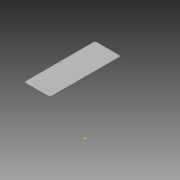
# Autodesk Inventor part: Base
Saved by Autodesk Inventor 2015 (Build 190159000, 159)
## iProperties
Created: 2014-07-24
Part Number: Base
Material: Generic
Document SubType Name: Modeling
Designer: Michael
Density: 1 g/cm^3
Appearance: Default
Author: Michael
Autodesk Inventor part; units mm, degrees
(part 1 of 2)
ref_plane "YZ Plane" through (0, 0, 0) normal (1, 0, 0) x (0, 1, 0)
ref_plane "XZ Plane" through (0, 0, 0) normal (0, 1, 0) x (-1, 0, 0)
ref_plane "XY Plane" through (0, 0, 0) normal (0, 0, 1) x (1, 0, 0)
sketch "Sketch1" plane through (0, 0, 0) normal (0, 1, 0) x (-1, 0, 0)
  circle A0 centre (194.2191, -316.0168) radius 1.4732
  circle A1 centre (279.9441, -316.0168) radius 1.4732
  circle A2 centre (279.9441, -192.1918) radius 1.4732
  circle A3 centre (194.2191, -192.1918) radius 1.4732
  circle A4 centre (194.2191, -68.3668) radius 1.4732
  circle A5 centre (279.9441, -68.3668) radius 1.4732
  arc A6 (191.0441, -316.0168) -> (194.2191, -319.1918) centre (194.2191, -316.0168) ccw
  arc A7 (279.9441, -319.1918) -> (283.1191, -316.0168) centre (279.9441, -316.0168) ccw
  arc A8 (194.2191, -65.1918) -> (191.0441, -68.3668) centre (194.2191, -68.3668) ccw
  arc A9 (283.1191, -68.3668) -> (279.9441, -65.1918) centre (279.9441, -68.3668) ccw
  line L0 (194.2191, -65.1918) -> (279.9441, -65.1918)
  line L1 (191.0441, -316.0168) -> (191.0441, -68.3668)
  line L2 (279.9441, -319.1918) -> (194.2191, -319.1918)
  line L3 (283.1191, -68.3668) -> (283.1191, -316.0168)
  circle A10 centre (95.0063, -316.0168) radius 1.4732
  circle A11 centre (180.7313, -316.0168) radius 1.4732
  circle A12 centre (180.7313, -192.1918) radius 1.4732
  circle A13 centre (95.0063, -192.1918) radius 1.4732
  circle A14 centre (95.0063, -68.3668) radius 1.4732
  circle A15 centre (180.7313, -68.3668) radius 1.4732
  arc A16 (91.8313, -316.0168) -> (95.0063, -319.1918) centre (95.0063, -316.0168) ccw
  arc A17 (180.7313, -319.1918) -> (183.9063, -316.0168) centre (180.7313, -316.0168) ccw
  line L4 (183.9063, -312.8418) -> (183.9063, -316.0168)
  line L5 (180.7313, -319.1918) -> (177.5563, -319.1918)
  arc A18 (95.0063, -65.1918) -> (91.8313, -68.3668) centre (95.0063, -68.3668) ccw
  line L6 (91.8313, -71.5418) -> (91.8313, -68.3668)
  line L7 (95.0063, -65.1918) -> (98.1813, -65.1918)
  arc A19 (183.9063, -68.3668) -> (180.7313, -65.1918) centre (180.7313, -68.3668) ccw
  line L8 (98.1813, -319.1918) -> (95.0063, -319.1918)
  line L9 (91.8313, -316.0168) -> (91.8313, -312.8418)
  line L10 (95.0063, -65.1918) -> (180.7313, -65.1918)
  line L11 (91.8313, -316.0168) -> (91.8313, -68.3668)
  line L12 (180.7313, -319.1918) -> (95.0063, -319.1918)
  line L13 (183.9063, -68.3668) -> (183.9063, -316.0168)
  line L14 (115.5168, -195.2716) -> (114.9834, -195.2716)
  line L15 (114.9834, -195.2716) -> (114.9834, -193.5952)
  line L16 (114.9834, -193.5952) -> (111.5798, -193.5952)
  line L17 (111.5798, -193.5952) -> (111.5798, -192.7062)
  line L18 (111.5798, -192.7062) -> (108.7858, -192.7062)
  line L19 (108.7858, -192.7062) -> (108.7858, -193.5952)
  line L20 (108.7858, -193.5952) -> (102.6898, -193.5952)
  line L21 (102.6898, -193.5952) -> (102.6898, -195.2716)
  line L22 (102.6898, -195.2716) -> (101.5468, -195.2716)
  line L23 (101.5468, -195.2716) -> (101.5468, -198.5736)
  line L24 (101.5468, -198.5736) -> (102.6898, -198.5736)
  line L25 (102.6898, -198.5736) -> (102.6898, -200.25)
  line L26 (102.6898, -200.25) -> (108.7858, -200.25)
  line L27 (108.7858, -200.25) -> (108.7858, -201.8756)
  line L28 (108.7858, -201.8756) -> (106.7894, -201.8756)
  line L29 (106.7894, -201.8756) -> (106.7894, -201.0628)
  line L30 (106.7894, -201.0628) -> (103.4772, -201.0628)
  line L31 (103.4772, -201.0628) -> (103.4772, -201.8756)
  line L32 (102.3088, -201.8756) -> (103.4772, -201.8756)
  line L33 (102.3088, -201.8756) -> (102.3088, -215.8456)
  line L34 (102.3088, -215.8456) -> (103.4772, -215.8456)
  line L35 (103.4772, -215.8456) -> (103.4772, -216.6584)
  line L36 (103.4772, -216.6584) -> (106.7894, -216.6584)
  line L37 (106.7894, -216.6584) -> (106.7894, -215.8456)
  line L38 (106.7894, -215.8456) -> (108.7858, -215.8456)
  line L39 (108.7858, -215.8456) -> (108.7858, -217.4712)
  line L40 (108.7858, -217.4712) -> (102.6898, -217.4712)
  line L41 (102.6898, -217.4712) -> (102.6898, -219.1476)
  line L42 (102.6898, -219.1476) -> (101.5468, -219.1476)
  line L43 (101.5468, -219.1476) -> (101.5468, -222.4496)
  line L44 (101.5468, -222.4496) -> (102.6898, -222.4496)
  line L45 (102.6898, -222.4496) -> (102.6898, -224.126)
  line L46 (102.6898, -224.126) -> (108.7858, -224.126)
  line L47 (108.7858, -224.126) -> (108.7858, -225.015)
  line L48 (108.7858, -225.015) -> (111.5798, -225.015)
  line L49 (111.5798, -225.015) -> (111.5798, -224.126)
  line L50 (111.5798, -224.126) -> (114.9834, -224.126)
  line L51 (114.9834, -224.126) -> (114.9834, -222.4496)
  line L52 (114.9834, -222.4496) -> (115.5168, -222.4496)
  line L53 (115.5168, -222.4496) -> (115.5168, -219.1476)
  line L54 (115.5168, -219.1476) -> (114.9834, -219.1476)
  line L55 (114.9834, -219.1476) -> (114.9834, -217.4712)
  line L56 (114.9834, -217.4712) -> (111.5798, -217.4712)
  line L57 (111.5798, -217.4712) -> (111.5798, -216.6584)
  line L58 (111.5798, -216.6584) -> (115.2984, -216.6584)
  line L59 (115.2984, -216.6584) -> (115.2984, -215.8456)
  line L60 (115.2984, -215.8456) -> (116.2788, -215.8456)
  line L61 (116.2788, -215.8456) -> (116.2788, -201.8756)
  line L62 (116.2788, -201.8756) -> (115.2984, -201.8756)
  line L63 (115.2984, -201.8756) -> (115.2984, -201.0628)
  line L64 (115.2984, -201.0628) -> (111.5798, -201.0628)
  line L65 (111.5798, -201.0628) -> (111.5798, -200.25)
  line L66 (111.5798, -200.25) -> (114.9834, -200.25)
  line L67 (114.9834, -200.25) -> (114.9834, -198.5736)
  line L68 (114.9834, -198.5736) -> (115.5168, -198.5736)
  line L69 (115.5168, -198.5736) -> (115.5168, -195.2716)
  line L70 (115.5168, -152.4091) -> (114.9834, -152.4091)
  line L71 (114.9834, -152.4091) -> (114.9834, -150.7327)
  line L72 (114.9834, -150.7327) -> (111.5798, -150.7327)
  line L73 (111.5798, -150.7327) -> (111.5798, -149.8437)
  line L74 (111.5798, -149.8437) -> (108.7858, -149.8437)
  line L75 (108.7858, -149.8437) -> (108.7858, -150.7327)
  line L76 (108.7858, -150.7327) -> (102.6898, -150.7327)
  line L77 (102.6898, -150.7327) -> (102.6898, -152.4091)
  line L78 (102.6898, -152.4091) -> (101.5468, -152.4091)
  line L79 (101.5468, -152.4091) -> (101.5468, -155.7111)
  line L80 (101.5468, -155.7111) -> (102.6898, -155.7111)
  line L81 (102.6898, -155.7111) -> (102.6898, -157.3875)
  line L82 (102.6898, -157.3875) -> (108.7858, -157.3875)
  line L83 (108.7858, -157.3875) -> (108.7858, -159.0131)
  line L84 (108.7858, -159.0131) -> (106.7894, -159.0131)
  line L85 (106.7894, -159.0131) -> (106.7894, -158.2003)
  line L86 (106.7894, -158.2003) -> (103.4772, -158.2003)
  line L87 (103.4772, -158.2003) -> (103.4772, -159.0131)
  line L88 (102.3088, -159.0131) -> (103.4772, -159.0131)
  line L89 (102.3088, -159.0131) -> (102.3088, -172.9831)
  line L90 (102.3088, -172.9831) -> (103.4772, -172.9831)
  line L91 (103.4772, -172.9831) -> (103.4772, -173.7959)
  line L92 (103.4772, -173.7959) -> (106.7894, -173.7959)
  line L93 (106.7894, -173.7959) -> (106.7894, -172.9831)
  line L94 (106.7894, -172.9831) -> (108.7858, -172.9831)
  line L95 (108.7858, -172.9831) -> (108.7858, -174.6087)
  line L96 (108.7858, -174.6087) -> (102.6898, -174.6087)
  line L97 (102.6898, -174.6087) -> (102.6898, -176.2851)
  line L98 (102.6898, -176.2851) -> (101.5468, -176.2851)
  line L99 (101.5468, -176.2851) -> (101.5468, -179.5871)
  line L100 (101.5468, -179.5871) -> (102.6898, -179.5871)
  line L101 (102.6898, -179.5871) -> (102.6898, -181.2635)
  line L102 (102.6898, -181.2635) -> (108.7858, -181.2635)
  line L103 (108.7858, -181.2635) -> (108.7858, -182.1525)
  line L104 (108.7858, -182.1525) -> (111.5798, -182.1525)
  line L105 (111.5798, -182.1525) -> (111.5798, -181.2635)
  line L106 (111.5798, -181.2635) -> (114.9834, -181.2635)
  line L107 (114.9834, -181.2635) -> (114.9834, -179.5871)
  line L108 (114.9834, -179.5871) -> (115.5168, -179.5871)
  line L109 (115.5168, -179.5871) -> (115.5168, -176.2851)
  line L110 (115.5168, -176.2851) -> (114.9834, -176.2851)
  line L111 (114.9834, -176.2851) -> (114.9834, -174.6087)
  line L112 (114.9834, -174.6087) -> (111.5798, -174.6087)
  line L113 (111.5798, -174.6087) -> (111.5798, -173.7959)
  line L114 (111.5798, -173.7959) -> (115.2984, -173.7959)
  line L115 (115.2984, -173.7959) -> (115.2984, -172.9831)
  line L116 (115.2984, -172.9831) -> (116.2788, -172.9831)
  line L117 (116.2788, -172.9831) -> (116.2788, -159.0131)
  line L118 (116.2788, -159.0131) -> (115.2984, -159.0131)
  line L119 (115.2984, -159.0131) -> (115.2984, -158.2003)
  line L120 (115.2984, -158.2003) -> (111.5798, -158.2003)
  line L121 (111.5798, -158.2003) -> (111.5798, -157.3875)
  line L122 (111.5798, -157.3875) -> (114.9834, -157.3875)
  line L123 (114.9834, -157.3875) -> (114.9834, -155.7111)
  line L124 (114.9834, -155.7111) -> (115.5168, -155.7111)
  line L125 (115.5168, -155.7111) -> (115.5168, -152.4091)
  line L126 (111.7982, -274.8815) -> (115.2983, -274.8815)
  line L127 (115.2983, -290.4771) -> (111.7982, -290.4771)
  line L128 (106.7893, -290.4771) -> (103.2892, -290.4771)
  line L129 (103.2892, -274.8815) -> (106.7893, -274.8815)
  line L130 (111.7982, -274.8815) -> (111.7982, -275.6943)
  line L131 (111.7982, -289.6643) -> (111.7982, -290.4771)
  line L132 (106.7893, -290.4771) -> (106.7893, -289.6643)
  line L133 (106.7893, -275.6943) -> (106.7893, -274.8815)
  line L134 (106.7893, -289.6643) -> (106.7893, -290.4771)
  line L135 (106.7893, -290.4771) -> (103.2892, -290.4771)
  line L136 (103.2892, -290.4771) -> (103.2892, -289.6643)
  line L137 (103.2892, -275.6943) -> (103.2892, -274.8815)
  line L138 (103.2892, -274.8815) -> (106.7893, -274.8815)
  line L139 (106.7893, -274.8815) -> (106.7893, -275.6943)
  line L140 (111.7982, -275.6943) -> (111.7982, -274.8815)
  line L141 (111.7982, -274.8815) -> (115.2983, -274.8815)
  line L142 (115.2983, -274.8815) -> (115.2983, -275.6943)
  line L143 (115.2983, -289.6643) -> (115.2983, -290.4771)
  line L144 (115.2983, -290.4771) -> (111.7982, -290.4771)
  line L145 (111.7982, -290.4771) -> (111.7982, -289.6643)
  line L146 (115.2983, -275.6943) -> (116.2788, -275.6943)
  line L147 (116.2788, -275.6943) -> (116.2788, -289.6643)
  line L148 (116.2788, -289.6643) -> (115.2983, -289.6643)
  line L149 (111.7982, -289.6643) -> (106.7893, -289.6643)
  line L150 (103.2892, -289.6643) -> (102.3088, -289.6643)
  line L151 (102.3088, -289.6643) -> (102.3088, -275.6943)
  line L152 (102.3088, -275.6943) -> (103.2892, -275.6943)
  line L153 (106.7893, -275.6943) -> (111.7982, -275.6943)
  line L154 (111.7982, -293.9315) -> (115.2983, -293.9315)
  line L155 (115.2983, -309.5271) -> (111.7982, -309.5271)
  line L156 (106.7893, -309.5271) -> (103.2892, -309.5271)
  line L157 (103.2892, -293.9315) -> (106.7893, -293.9315)
  line L158 (111.7982, -293.9315) -> (111.7982, -294.7443)
  line L159 (111.7982, -308.7143) -> (111.7982, -309.5271)
  line L160 (106.7893, -309.5271) -> (106.7893, -308.7143)
  line L161 (106.7893, -294.7443) -> (106.7893, -293.9315)
  line L162 (106.7893, -308.7143) -> (106.7893, -309.5271)
  line L163 (106.7893, -309.5271) -> (103.2892, -309.5271)
  line L164 (103.2892, -309.5271) -> (103.2892, -308.7143)
  line L165 (103.2892, -294.7443) -> (103.2892, -293.9315)
  line L166 (103.2892, -293.9315) -> (106.7893, -293.9315)
  line L167 (106.7893, -293.9315) -> (106.7893, -294.7443)
  line L168 (111.7982, -294.7443) -> (111.7982, -293.9315)
  line L169 (111.7982, -293.9315) -> (115.2983, -293.9315)
  line L170 (115.2983, -293.9315) -> (115.2983, -294.7443)
  line L171 (115.2983, -308.7143) -> (115.2983, -309.5271)
  line L172 (115.2983, -309.5271) -> (111.7982, -309.5271)
  line L173 (111.7982, -309.5271) -> (111.7982, -308.7143)
  line L174 (115.2983, -294.7443) -> (116.2788, -294.7443)
  line L175 (116.2788, -294.7443) -> (116.2788, -308.7143)
  line L176 (116.2788, -308.7143) -> (115.2983, -308.7143)
  line L177 (111.7982, -308.7143) -> (106.7893, -308.7143)
  line L178 (103.2892, -308.7143) -> (102.3088, -308.7143)
  line L179 (102.3088, -308.7143) -> (102.3088, -294.7443)
  line L180 (102.3088, -294.7443) -> (103.2892, -294.7443)
  line L181 (106.7893, -294.7443) -> (111.7982, -294.7443)
  line L182 (111.7982, -255.8315) -> (115.2983, -255.8315)
  line L183 (115.2983, -271.4271) -> (111.7982, -271.4271)
  line L184 (106.7893, -271.4271) -> (103.2892, -271.4271)
  line L185 (103.2892, -255.8315) -> (106.7893, -255.8315)
  line L186 (111.7982, -255.8315) -> (111.7982, -256.6443)
  line L187 (111.7982, -270.6143) -> (111.7982, -271.4271)
  line L188 (106.7893, -271.4271) -> (106.7893, -270.6143)
  line L189 (106.7893, -256.6443) -> (106.7893, -255.8315)
  line L190 (106.7893, -270.6143) -> (106.7893, -271.4271)
  line L191 (106.7893, -271.4271) -> (103.2892, -271.4271)
  line L192 (103.2892, -271.4271) -> (103.2892, -270.6143)
  line L193 (103.2892, -256.6443) -> (103.2892, -255.8315)
  line L194 (103.2892, -255.8315) -> (106.7893, -255.8315)
  line L195 (106.7893, -255.8315) -> (106.7893, -256.6443)
  line L196 (111.7982, -256.6443) -> (111.7982, -255.8315)
  line L197 (111.7982, -255.8315) -> (115.2983, -255.8315)
  line L198 (115.2983, -255.8315) -> (115.2983, -256.6443)
  line L199 (115.2983, -270.6143) -> (115.2983, -271.4271)
  line L200 (115.2983, -271.4271) -> (111.7982, -271.4271)
  line L201 (111.7982, -271.4271) -> (111.7982, -270.6143)
  line L202 (115.2983, -256.6443) -> (116.2788, -256.6443)
  line L203 (116.2788, -256.6443) -> (116.2788, -270.6143)
  line L204 (116.2788, -270.6143) -> (115.2983, -270.6143)
  line L205 (111.7982, -270.6143) -> (106.7893, -270.6143)
  line L206 (103.2892, -270.6143) -> (102.3088, -270.6143)
  line L207 (102.3088, -270.6143) -> (102.3088, -256.6443)
  line L208 (102.3088, -256.6443) -> (103.2892, -256.6443)
  line L209 (106.7893, -256.6443) -> (111.7982, -256.6443)
  line L210 (111.7982, -234.4003) -> (115.2983, -234.4003)
  line L211 (115.2983, -249.9959) -> (111.7982, -249.9959)
  line L212 (106.7893, -249.9959) -> (103.2892, -249.9959)
  line L213 (103.2892, -234.4003) -> (106.7893, -234.4003)
  line L214 (111.7982, -234.4003) -> (111.7982, -235.2131)
  line L215 (111.7982, -249.1831) -> (111.7982, -249.9959)
  line L216 (106.7893, -249.9959) -> (106.7893, -249.1831)
  line L217 (106.7893, -235.2131) -> (106.7893, -234.4003)
  line L218 (106.7893, -249.1831) -> (106.7893, -249.9959)
  line L219 (106.7893, -249.9959) -> (103.2892, -249.9959)
  line L220 (103.2892, -249.9959) -> (103.2892, -249.1831)
  line L221 (103.2892, -235.2131) -> (103.2892, -234.4003)
  line L222 (103.2892, -234.4003) -> (106.7893, -234.4003)
  line L223 (106.7893, -234.4003) -> (106.7893, -235.2131)
  line L224 (111.7982, -235.2131) -> (111.7982, -234.4003)
  line L225 (111.7982, -234.4003) -> (115.2983, -234.4003)
  line L226 (115.2983, -234.4003) -> (115.2983, -235.2131)
  line L227 (115.2983, -249.1831) -> (115.2983, -249.9959)
  line L228 (115.2983, -249.9959) -> (111.7982, -249.9959)
  line L229 (111.7982, -249.9959) -> (111.7982, -249.1831)
  line L230 (115.2983, -235.2131) -> (116.2788, -235.2131)
  line L231 (116.2788, -235.2131) -> (116.2788, -249.1831)
  line L232 (116.2788, -249.1831) -> (115.2983, -249.1831)
  line L233 (111.7982, -249.1831) -> (106.7893, -249.1831)
  line L234 (103.2892, -249.1831) -> (102.3088, -249.1831)
  line L235 (102.3088, -249.1831) -> (102.3088, -235.2131)
  line L236 (102.3088, -235.2131) -> (103.2892, -235.2131)
  line L237 (106.7893, -235.2131) -> (111.7982, -235.2131)
  line L238 (111.7982, -101.0503) -> (115.2983, -101.0503)
  line L239 (115.2983, -116.6459) -> (111.7982, -116.6459)
  line L240 (106.7893, -116.6459) -> (103.2892, -116.6459)
  line L241 (103.2892, -101.0503) -> (106.7893, -101.0503)
  line L242 (111.7982, -101.0503) -> (111.7982, -101.8631)
  line L243 (111.7982, -115.8331) -> (111.7982, -116.6459)
  line L244 (106.7893, -116.6459) -> (106.7893, -115.8331)
  line L245 (106.7893, -101.8631) -> (106.7893, -101.0503)
  line L246 (106.7893, -115.8331) -> (106.7893, -116.6459)
  line L247 (106.7893, -116.6459) -> (103.2892, -116.6459)
  line L248 (103.2892, -116.6459) -> (103.2892, -115.8331)
  line L249 (103.2892, -101.8631) -> (103.2892, -101.0503)
  line L250 (103.2892, -101.0503) -> (106.7893, -101.0503)
  line L251 (106.7893, -101.0503) -> (106.7893, -101.8631)
  line L252 (111.7982, -101.8631) -> (111.7982, -101.0503)
  line L253 (111.7982, -101.0503) -> (115.2983, -101.0503)
  line L254 (115.2983, -101.0503) -> (115.2983, -101.8631)
  line L255 (115.2983, -115.8331) -> (115.2983, -116.6459)
  line L256 (115.2983, -116.6459) -> (111.7982, -116.6459)
  line L257 (111.7982, -116.6459) -> (111.7982, -115.8331)
  line L258 (115.2983, -101.8631) -> (116.2788, -101.8631)
  line L259 (116.2788, -101.8631) -> (116.2788, -115.8331)
  line L260 (116.2788, -115.8331) -> (115.2983, -115.8331)
  line L261 (111.7982, -115.8331) -> (106.7893, -115.8331)
  line L262 (103.2892, -115.8331) -> (102.3088, -115.8331)
  line L263 (102.3088, -115.8331) -> (102.3088, -101.8631)
  line L264 (102.3088, -101.8631) -> (103.2892, -101.8631)
  line L265 (106.7893, -101.8631) -> (111.7982, -101.8631)
  line L266 (111.7982, -124.8628) -> (115.2983, -124.8628)
  line L267 (115.2983, -140.4584) -> (111.7982, -140.4584)
  line L268 (106.7893, -140.4584) -> (103.2892, -140.4584)
  line L269 (103.2892, -124.8628) -> (106.7893, -124.8628)
  line L270 (111.7982, -124.8628) -> (111.7982, -125.6756)
  line L271 (111.7982, -139.6456) -> (111.7982, -140.4584)
  line L272 (106.7893, -140.4584) -> (106.7893, -139.6456)
  line L273 (106.7893, -125.6756) -> (106.7893, -124.8628)
  line L274 (106.7893, -139.6456) -> (106.7893, -140.4584)
  line L275 (106.7893, -140.4584) -> (103.2892, -140.4584)
  line L276 (103.2892, -140.4584) -> (103.2892, -139.6456)
  line L277 (103.2892, -125.6756) -> (103.2892, -124.8628)
  line L278 (103.2892, -124.8628) -> (106.7893, -124.8628)
  line L279 (106.7893, -124.8628) -> (106.7893, -125.6756)
  line L280 (111.7982, -125.6756) -> (111.7982, -124.8628)
  line L281 (111.7982, -124.8628) -> (115.2983, -124.8628)
  line L282 (115.2983, -124.8628) -> (115.2983, -125.6756)
  line L283 (115.2983, -139.6456) -> (115.2983, -140.4584)
  line L284 (115.2983, -140.4584) -> (111.7982, -140.4584)
  line L285 (111.7982, -140.4584) -> (111.7982, -139.6456)
  line L286 (115.2983, -125.6756) -> (116.2788, -125.6756)
  line L287 (116.2788, -125.6756) -> (116.2788, -139.6456)
  line L288 (116.2788, -139.6456) -> (115.2983, -139.6456)
  line L289 (111.7982, -139.6456) -> (106.7893, -139.6456)
  line L290 (103.2892, -139.6456) -> (102.3088, -139.6456)
  line L291 (102.3088, -139.6456) -> (102.3088, -125.6756)
  line L292 (102.3088, -125.6756) -> (103.2892, -125.6756)
  line L293 (106.7893, -125.6756) -> (111.7982, -125.6756)
  line L294 (111.7982, -77.2378) -> (115.2983, -77.2378)
  line L295 (115.2983, -92.8334) -> (111.7982, -92.8334)
  line L296 (106.7893, -92.8334) -> (103.2892, -92.8334)
  line L297 (103.2892, -77.2378) -> (106.7893, -77.2378)
  line L298 (111.7982, -77.2378) -> (111.7982, -78.0506)
  line L299 (111.7982, -92.0206) -> (111.7982, -92.8334)
  line L300 (106.7893, -92.8334) -> (106.7893, -92.0206)
  line L301 (106.7893, -78.0506) -> (106.7893, -77.2378)
  line L302 (106.7893, -92.0206) -> (106.7893, -92.8334)
  line L303 (106.7893, -92.8334) -> (103.2892, -92.8334)
  line L304 (103.2892, -92.8334) -> (103.2892, -92.0206)
  line L305 (103.2892, -78.0506) -> (103.2892, -77.2378)
  line L306 (103.2892, -77.2378) -> (106.7893, -77.2378)
  line L307 (106.7893, -77.2378) -> (106.7893, -78.0506)
  line L308 (111.7982, -78.0506) -> (111.7982, -77.2378)
  line L309 (111.7982, -77.2378) -> (115.2983, -77.2378)
  line L310 (115.2983, -77.2378) -> (115.2983, -78.0506)
  line L311 (115.2983, -92.0206) -> (115.2983, -92.8334)
  line L312 (115.2983, -92.8334) -> (111.7982, -92.8334)
  line L313 (111.7982, -92.8334) -> (111.7982, -92.0206)
  line L314 (115.2983, -78.0506) -> (116.2788, -78.0506)
  line L315 (116.2788, -78.0506) -> (116.2788, -92.0206)
  line L316 (116.2788, -92.0206) -> (115.2983, -92.0206)
  line L317 (111.7982, -92.0206) -> (106.7893, -92.0206)
  line L318 (103.2892, -92.0206) -> (102.3088, -92.0206)
  line L319 (102.3088, -92.0206) -> (102.3088, -78.0506)
  line L320 (102.3088, -78.0506) -> (103.2892, -78.0506)
  line L321 (106.7893, -78.0506) -> (111.7982, -78.0506)
  line L322 (130.8482, -122.4815) -> (134.3483, -122.4815)
  line L323 (134.3483, -138.0771) -> (130.8482, -138.0771)
  line L324 (125.8393, -138.0771) -> (122.3392, -138.0771)
  line L325 (122.3392, -122.4815) -> (125.8393, -122.4815)
  line L326 (130.8482, -122.4815) -> (130.8482, -123.2943)
  line L327 (130.8482, -137.2643) -> (130.8482, -138.0771)
  line L328 (125.8393, -138.0771) -> (125.8393, -137.2643)
  line L329 (125.8393, -123.2943) -> (125.8393, -122.4815)
  line L330 (125.8393, -137.2643) -> (125.8393, -138.0771)
  line L331 (125.8393, -138.0771) -> (122.3392, -138.0771)
  line L332 (122.3392, -138.0771) -> (122.3392, -137.2643)
  line L333 (122.3392, -123.2943) -> (122.3392, -122.4815)
  line L334 (122.3392, -122.4815) -> (125.8393, -122.4815)
  line L335 (125.8393, -122.4815) -> (125.8393, -123.2943)
  line L336 (130.8482, -123.2943) -> (130.8482, -122.4815)
  line L337 (130.8482, -122.4815) -> (134.3483, -122.4815)
  line L338 (134.3483, -122.4815) -> (134.3483, -123.2943)
  line L339 (134.3483, -137.2643) -> (134.3483, -138.0771)
  line L340 (134.3483, -138.0771) -> (130.8482, -138.0771)
  line L341 (130.8482, -138.0771) -> (130.8482, -137.2643)
  line L342 (134.3483, -123.2943) -> (135.3288, -123.2943)
  line L343 (135.3288, -123.2943) -> (135.3288, -137.2643)
  line L344 (135.3288, -137.2643) -> (134.3483, -137.2643)
  line L345 (130.8482, -137.2643) -> (125.8393, -137.2643)
  line L346 (122.3392, -137.2643) -> (121.3588, -137.2643)
  line L347 (121.3588, -137.2643) -> (121.3588, -123.2943)
  line L348 (121.3588, -123.2943) -> (122.3392, -123.2943)
  line L349 (125.8393, -123.2943) -> (130.8482, -123.2943)
  line L350 (130.8482, -141.5315) -> (134.3483, -141.5315)
  line L351 (134.3483, -157.1271) -> (130.8482, -157.1271)
  line L352 (125.8393, -157.1271) -> (122.3392, -157.1271)
  line L353 (122.3392, -141.5315) -> (125.8393, -141.5315)
  line L354 (130.8482, -141.5315) -> (130.8482, -142.3443)
  line L355 (130.8482, -156.3143) -> (130.8482, -157.1271)
  line L356 (125.8393, -157.1271) -> (125.8393, -156.3143)
  line L357 (125.8393, -142.3443) -> (125.8393, -141.5315)
  line L358 (125.8393, -156.3143) -> (125.8393, -157.1271)
  line L359 (125.8393, -157.1271) -> (122.3392, -157.1271)
  line L360 (122.3392, -157.1271) -> (122.3392, -156.3143)
  line L361 (122.3392, -142.3443) -> (122.3392, -141.5315)
  line L362 (122.3392, -141.5315) -> (125.8393, -141.5315)
  line L363 (125.8393, -141.5315) -> (125.8393, -142.3443)
  line L364 (130.8482, -142.3443) -> (130.8482, -141.5315)
  line L365 (130.8482, -141.5315) -> (134.3483, -141.5315)
  line L366 (134.3483, -141.5315) -> (134.3483, -142.3443)
  line L367 (134.3483, -156.3143) -> (134.3483, -157.1271)
  line L368 (134.3483, -157.1271) -> (130.8482, -157.1271)
  line L369 (130.8482, -157.1271) -> (130.8482, -156.3143)
  line L370 (134.3483, -142.3443) -> (135.3288, -142.3443)
  line L371 (135.3288, -142.3443) -> (135.3288, -156.3143)
  line L372 (135.3288, -156.3143) -> (134.3483, -156.3143)
  line L373 (130.8482, -156.3143) -> (125.8393, -156.3143)
  line L374 (122.3392, -156.3143) -> (121.3588, -156.3143)
  line L375 (121.3588, -156.3143) -> (121.3588, -142.3443)
  line L376 (121.3588, -142.3443) -> (122.3392, -142.3443)
  line L377 (125.8393, -142.3443) -> (130.8482, -142.3443)
  line L378 (130.8482, -160.5815) -> (134.3483, -160.5815)
  line L379 (134.3483, -176.1771) -> (130.8482, -176.1771)
  line L380 (125.8393, -176.1771) -> (122.3392, -176.1771)
  line L381 (122.3392, -160.5815) -> (125.8393, -160.5815)
  line L382 (130.8482, -160.5815) -> (130.8482, -161.3943)
  line L383 (130.8482, -175.3643) -> (130.8482, -176.1771)
  line L384 (125.8393, -176.1771) -> (125.8393, -175.3643)
  line L385 (125.8393, -161.3943) -> (125.8393, -160.5815)
  line L386 (125.8393, -175.3643) -> (125.8393, -176.1771)
  line L387 (125.8393, -176.1771) -> (122.3392, -176.1771)
  line L388 (122.3392, -176.1771) -> (122.3392, -175.3643)
  line L389 (122.3392, -161.3943) -> (122.3392, -160.5815)
  line L390 (122.3392, -160.5815) -> (125.8393, -160.5815)
  line L391 (125.8393, -160.5815) -> (125.8393, -161.3943)
  line L392 (130.8482, -161.3943) -> (130.8482, -160.5815)
  line L393 (130.8482, -160.5815) -> (134.3483, -160.5815)
  line L394 (134.3483, -160.5815) -> (134.3483, -161.3943)
  line L395 (134.3483, -175.3643) -> (134.3483, -176.1771)
  line L396 (134.3483, -176.1771) -> (130.8482, -176.1771)
  line L397 (130.8482, -176.1771) -> (130.8482, -175.3643)
  line L398 (134.3483, -161.3943) -> (135.3288, -161.3943)
  line L399 (135.3288, -161.3943) -> (135.3288, -175.3643)
  line L400 (135.3288, -175.3643) -> (134.3483, -175.3643)
  line L401 (130.8482, -175.3643) -> (125.8393, -175.3643)
  line L402 (122.3392, -175.3643) -> (121.3588, -175.3643)
  line L403 (121.3588, -175.3643) -> (121.3588, -161.3943)
  line L404 (121.3588, -161.3943) -> (122.3392, -161.3943)
  line L405 (125.8393, -161.3943) -> (130.8482, -161.3943)
  line L406 (130.8482, -179.6315) -> (134.3483, -179.6315)
  line L407 (134.3483, -195.2271) -> (130.8482, -195.2271)
  line L408 (125.8393, -195.2271) -> (122.3392, -195.2271)
  line L409 (122.3392, -179.6315) -> (125.8393, -179.6315)
  line L410 (130.8482, -179.6315) -> (130.8482, -180.4443)
  line L411 (130.8482, -194.4143) -> (130.8482, -195.2271)
  line L412 (125.8393, -195.2271) -> (125.8393, -194.4143)
  line L413 (125.8393, -180.4443) -> (125.8393, -179.6315)
  line L414 (125.8393, -194.4143) -> (125.8393, -195.2271)
  line L415 (125.8393, -195.2271) -> (122.3392, -195.2271)
  line L416 (122.3392, -195.2271) -> (122.3392, -194.4143)
  line L417 (122.3392, -180.4443) -> (122.3392, -179.6315)
  line L418 (122.3392, -179.6315) -> (125.8393, -179.6315)
  line L419 (125.8393, -179.6315) -> (125.8393, -180.4443)
  line L420 (130.8482, -180.4443) -> (130.8482, -179.6315)
  line L421 (130.8482, -179.6315) -> (134.3483, -179.6315)
  line L422 (134.3483, -179.6315) -> (134.3483, -180.4443)
  line L423 (134.3483, -194.4143) -> (134.3483, -195.2271)
  line L424 (134.3483, -195.2271) -> (130.8482, -195.2271)
  line L425 (130.8482, -195.2271) -> (130.8482, -194.4143)
  line L426 (134.3483, -180.4443) -> (135.3288, -180.4443)
  line L427 (135.3288, -180.4443) -> (135.3288, -194.4143)
  line L428 (135.3288, -194.4143) -> (134.3483, -194.4143)
  line L429 (130.8482, -194.4143) -> (125.8393, -194.4143)
  line L430 (122.3392, -194.4143) -> (121.3588, -194.4143)
  line L431 (121.3588, -194.4143) -> (121.3588, -180.4443)
  line L432 (121.3588, -180.4443) -> (122.3392, -180.4443)
  line L433 (125.8393, -180.4443) -> (130.8482, -180.4443)
  line L434 (130.8482, -198.6815) -> (134.3483, -198.6815)
  line L435 (134.3483, -214.2771) -> (130.8482, -214.2771)
  line L436 (125.8393, -214.2771) -> (122.3392, -214.2771)
  line L437 (122.3392, -198.6815) -> (125.8393, -198.6815)
  line L438 (130.8482, -198.6815) -> (130.8482, -199.4943)
  line L439 (130.8482, -213.4643) -> (130.8482, -214.2771)
  line L440 (125.8393, -214.2771) -> (125.8393, -213.4643)
  line L441 (125.8393, -199.4943) -> (125.8393, -198.6815)
  line L442 (125.8393, -213.4643) -> (125.8393, -214.2771)
  line L443 (125.8393, -214.2771) -> (122.3392, -214.2771)
  line L444 (122.3392, -214.2771) -> (122.3392, -213.4643)
  line L445 (122.3392, -199.4943) -> (122.3392, -198.6815)
  line L446 (122.3392, -198.6815) -> (125.8393, -198.6815)
  line L447 (125.8393, -198.6815) -> (125.8393, -199.4943)
  line L448 (130.8482, -199.4943) -> (130.8482, -198.6815)
  line L449 (130.8482, -198.6815) -> (134.3483, -198.6815)
  line L450 (134.3483, -198.6815) -> (134.3483, -199.4943)
  line L451 (134.3483, -213.4643) -> (134.3483, -214.2771)
  line L452 (134.3483, -214.2771) -> (130.8482, -214.2771)
  line L453 (130.8482, -214.2771) -> (130.8482, -213.4643)
  line L454 (134.3483, -199.4943) -> (135.3288, -199.4943)
  line L455 (135.3288, -199.4943) -> (135.3288, -213.4643)
  line L456 (135.3288, -213.4643) -> (134.3483, -213.4643)
  line L457 (130.8482, -213.4643) -> (125.8393, -213.4643)
  line L458 (122.3392, -213.4643) -> (121.3588, -213.4643)
  line L459 (121.3588, -213.4643) -> (121.3588, -199.4943)
  line L460 (121.3588, -199.4943) -> (122.3392, -199.4943)
  line L461 (125.8393, -199.4943) -> (130.8482, -199.4943)
  line L462 (130.8482, -217.7315) -> (134.3483, -217.7315)
  line L463 (134.3483, -233.3271) -> (130.8482, -233.3271)
  line L464 (125.8393, -233.3271) -> (122.3392, -233.3271)
  line L465 (122.3392, -217.7315) -> (125.8393, -217.7315)
  line L466 (130.8482, -217.7315) -> (130.8482, -218.5443)
  line L467 (130.8482, -232.5143) -> (130.8482, -233.3271)
  line L468 (125.8393, -233.3271) -> (125.8393, -232.5143)
  line L469 (125.8393, -218.5443) -> (125.8393, -217.7315)
  line L470 (125.8393, -232.5143) -> (125.8393, -233.3271)
  line L471 (125.8393, -233.3271) -> (122.3392, -233.3271)
  line L472 (122.3392, -233.3271) -> (122.3392, -232.5143)
  line L473 (122.3392, -218.5443) -> (122.3392, -217.7315)
  line L474 (122.3392, -217.7315) -> (125.8393, -217.7315)
  line L475 (125.8393, -217.7315) -> (125.8393, -218.5443)
  line L476 (130.8482, -218.5443) -> (130.8482, -217.7315)
  line L477 (130.8482, -217.7315) -> (134.3483, -217.7315)
  line L478 (134.3483, -217.7315) -> (134.3483, -218.5443)
  line L479 (134.3483, -232.5143) -> (134.3483, -233.3271)
  line L480 (134.3483, -233.3271) -> (130.8482, -233.3271)
  line L481 (130.8482, -233.3271) -> (130.8482, -232.5143)
  line L482 (134.3483, -218.5443) -> (135.3288, -218.5443)
  line L483 (135.3288, -218.5443) -> (135.3288, -232.5143)
  line L484 (135.3288, -232.5143) -> (134.3483, -232.5143)
  line L485 (130.8482, -232.5143) -> (125.8393, -232.5143)
  line L486 (122.3392, -232.5143) -> (121.3588, -232.5143)
  line L487 (121.3588, -232.5143) -> (121.3588, -218.5443)
  line L488 (121.3588, -218.5443) -> (122.3392, -218.5443)
  line L489 (125.8393, -218.5443) -> (130.8482, -218.5443)
  line L490 (130.8482, -236.7815) -> (134.3483, -236.7815)
  line L491 (134.3483, -252.3771) -> (130.8482, -252.3771)
  line L492 (125.8393, -252.3771) -> (122.3392, -252.3771)
  line L493 (122.3392, -236.7815) -> (125.8393, -236.7815)
  line L494 (130.8482, -236.7815) -> (130.8482, -237.5943)
  line L495 (130.8482, -251.5643) -> (130.8482, -252.3771)
  line L496 (125.8393, -252.3771) -> (125.8393, -251.5643)
  line L497 (125.8393, -237.5943) -> (125.8393, -236.7815)
  line L498 (125.8393, -251.5643) -> (125.8393, -252.3771)
  line L499 (125.8393, -252.3771) -> (122.3392, -252.3771)
  line L500 (122.3392, -252.3771) -> (122.3392, -251.5643)
  line L501 (122.3392, -237.5943) -> (122.3392, -236.7815)
  line L502 (122.3392, -236.7815) -> (125.8393, -236.7815)
  line L503 (125.8393, -236.7815) -> (125.8393, -237.5943)
  line L504 (130.8482, -237.5943) -> (130.8482, -236.7815)
  line L505 (130.8482, -236.7815) -> (134.3483, -236.7815)
  line L506 (134.3483, -236.7815) -> (134.3483, -237.5943)
  line L507 (134.3483, -251.5643) -> (134.3483, -252.3771)
  line L508 (134.3483, -252.3771) -> (130.8482, -252.3771)
  line L509 (130.8482, -252.3771) -> (130.8482, -251.5643)
  line L510 (134.3483, -237.5943) -> (135.3288, -237.5943)
  line L511 (135.3288, -237.5943) -> (135.3288, -251.5643)
  line L512 (135.3288, -251.5643) -> (134.3483, -251.5643)
  line L513 (130.8482, -251.5643) -> (125.8393, -251.5643)
  line L514 (122.3392, -251.5643) -> (121.3588, -251.5643)
  line L515 (121.3588, -251.5643) -> (121.3588, -237.5943)
  line L516 (121.3588, -237.5943) -> (122.3392, -237.5943)
  line L517 (125.8393, -237.5943) -> (130.8482, -237.5943)
  line L518 (130.8482, -255.8315) -> (134.3483, -255.8315)
  line L519 (134.3483, -271.4271) -> (130.8482, -271.4271)
  line L520 (125.8393, -271.4271) -> (122.3392, -271.4271)
  line L521 (122.3392, -255.8315) -> (125.8393, -255.8315)
  line L522 (130.8482, -255.8315) -> (130.8482, -256.6443)
  line L523 (130.8482, -270.6143) -> (130.8482, -271.4271)
  line L524 (125.8393, -271.4271) -> (125.8393, -270.6143)
  line L525 (125.8393, -256.6443) -> (125.8393, -255.8315)
  line L526 (125.8393, -270.6143) -> (125.8393, -271.4271)
  line L527 (125.8393, -271.4271) -> (122.3392, -271.4271)
  line L528 (122.3392, -271.4271) -> (122.3392, -270.6143)
  line L529 (122.3392, -256.6443) -> (122.3392, -255.8315)
  line L530 (122.3392, -255.8315) -> (125.8393, -255.8315)
  line L531 (125.8393, -255.8315) -> (125.8393, -256.6443)
  line L532 (130.8482, -256.6443) -> (130.8482, -255.8315)
  line L533 (130.8482, -255.8315) -> (134.3483, -255.8315)
  line L534 (134.3483, -255.8315) -> (134.3483, -256.6443)
  line L535 (134.3483, -270.6143) -> (134.3483, -271.4271)
  line L536 (134.3483, -271.4271) -> (130.8482, -271.4271)
  line L537 (130.8482, -271.4271) -> (130.8482, -270.6143)
  line L538 (134.3483, -256.6443) -> (135.3288, -256.6443)
  line L539 (135.3288, -256.6443) -> (135.3288, -270.6143)
  line L540 (135.3288, -270.6143) -> (134.3483, -270.6143)
  line L541 (130.8482, -270.6143) -> (125.8393, -270.6143)
  line L542 (122.3392, -270.6143) -> (121.3588, -270.6143)
  line L543 (121.3588, -270.6143) -> (121.3588, -256.6443)
  line L544 (121.3588, -256.6443) -> (122.3392, -256.6443)
  line L545 (125.8393, -256.6443) -> (130.8482, -256.6443)
  line L546 (130.8482, -274.8815) -> (134.3483, -274.8815)
  line L547 (134.3483, -290.4771) -> (130.8482, -290.4771)
  line L548 (125.8393, -290.4771) -> (122.3392, -290.4771)
  line L549 (122.3392, -274.8815) -> (125.8393, -274.8815)
  line L550 (130.8482, -274.8815) -> (130.8482, -275.6943)
  line L551 (130.8482, -289.6643) -> (130.8482, -290.4771)
  line L552 (125.8393, -290.4771) -> (125.8393, -289.6643)
  line L553 (125.8393, -275.6943) -> (125.8393, -274.8815)
  line L554 (125.8393, -289.6643) -> (125.8393, -290.4771)
  line L555 (125.8393, -290.4771) -> (122.3392, -290.4771)
  line L556 (122.3392, -290.4771) -> (122.3392, -289.6643)
  line L557 (122.3392, -275.6943) -> (122.3392, -274.8815)
  line L558 (122.3392, -274.8815) -> (125.8393, -274.8815)
  line L559 (125.8393, -274.8815) -> (125.8393, -275.6943)
  line L560 (130.8482, -275.6943) -> (130.8482, -274.8815)
  line L561 (130.8482, -274.8815) -> (134.3483, -274.8815)
  line L562 (134.3483, -274.8815) -> (134.3483, -275.6943)
  line L563 (134.3483, -289.6643) -> (134.3483, -290.4771)
  line L564 (134.3483, -290.4771) -> (130.8482, -290.4771)
  line L565 (130.8482, -290.4771) -> (130.8482, -289.6643)
  line L566 (134.3483, -275.6943) -> (135.3288, -275.6943)
  line L567 (135.3288, -275.6943) -> (135.3288, -289.6643)
  line L568 (135.3288, -289.6643) -> (134.3483, -289.6643)
  line L569 (130.8482, -289.6643) -> (125.8393, -289.6643)
  line L570 (122.3392, -289.6643) -> (121.3588, -289.6643)
  line L571 (121.3588, -289.6643) -> (121.3588, -275.6943)
  line L572 (121.3588, -275.6943) -> (122.3392, -275.6943)
  line L573 (125.8393, -275.6943) -> (130.8482, -275.6943)
  line L574 (130.8482, -293.9315) -> (134.3483, -293.9315)
  line L575 (134.3483, -309.5271) -> (130.8482, -309.5271)
  line L576 (125.8393, -309.5271) -> (122.3392, -309.5271)
  line L577 (122.3392, -293.9315) -> (125.8393, -293.9315)
  line L578 (130.8482, -293.9315) -> (130.8482, -294.7443)
  line L579 (130.8482, -308.7143) -> (130.8482, -309.5271)
  line L580 (125.8393, -309.5271) -> (125.8393, -308.7143)
  line L581 (125.8393, -294.7443) -> (125.8393, -293.9315)
  line L582 (125.8393, -308.7143) -> (125.8393, -309.5271)
  line L583 (125.8393, -309.5271) -> (122.3392, -309.5271)
  line L584 (122.3392, -309.5271) -> (122.3392, -308.7143)
  line L585 (122.3392, -294.7443) -> (122.3392, -293.9315)
  line L586 (122.3392, -293.9315) -> (125.8393, -293.9315)
  line L587 (125.8393, -293.9315) -> (125.8393, -294.7443)
  line L588 (130.8482, -294.7443) -> (130.8482, -293.9315)
  line L589 (130.8482, -293.9315) -> (134.3483, -293.9315)
  line L590 (134.3483, -293.9315) -> (134.3483, -294.7443)
  line L591 (134.3483, -308.7143) -> (134.3483, -309.5271)
  line L592 (134.3483, -309.5271) -> (130.8482, -309.5271)
  line L593 (130.8482, -309.5271) -> (130.8482, -308.7143)
  line L594 (134.3483, -294.7443) -> (135.3288, -294.7443)
  line L595 (135.3288, -294.7443) -> (135.3288, -308.7143)
  line L596 (135.3288, -308.7143) -> (134.3483, -308.7143)
  line L597 (130.8482, -308.7143) -> (125.8393, -308.7143)
  line L598 (122.3392, -308.7143) -> (121.3588, -308.7143)
  line L599 (121.3588, -308.7143) -> (121.3588, -294.7443)
  line L600 (121.3588, -294.7443) -> (122.3392, -294.7443)
  line L601 (125.8393, -294.7443) -> (130.8482, -294.7443)
  line L602 (130.8482, -103.4315) -> (134.3483, -103.4315)
  line L603 (134.3483, -119.0271) -> (130.8482, -119.0271)
  line L604 (125.8393, -119.0271) -> (122.3392, -119.0271)
  line L605 (122.3392, -103.4315) -> (125.8393, -103.4315)
  line L606 (130.8482, -103.4315) -> (130.8482, -104.2443)
  line L607 (130.8482, -118.2143) -> (130.8482, -119.0271)
  line L608 (125.8393, -119.0271) -> (125.8393, -118.2143)
  line L609 (125.8393, -104.2443) -> (125.8393, -103.4315)
  line L610 (125.8393, -118.2143) -> (125.8393, -119.0271)
  line L611 (125.8393, -119.0271) -> (122.3392, -119.0271)
  line L612 (122.3392, -119.0271) -> (122.3392, -118.2143)
  line L613 (122.3392, -104.2443) -> (122.3392, -103.4315)
  line L614 (122.3392, -103.4315) -> (125.8393, -103.4315)
  line L615 (125.8393, -103.4315) -> (125.8393, -104.2443)
  line L616 (130.8482, -104.2443) -> (130.8482, -103.4315)
  line L617 (130.8482, -103.4315) -> (134.3483, -103.4315)
  line L618 (134.3483, -103.4315) -> (134.3483, -104.2443)
  line L619 (134.3483, -118.2143) -> (134.3483, -119.0271)
  line L620 (134.3483, -119.0271) -> (130.8482, -119.0271)
  line L621 (130.8482, -119.0271) -> (130.8482, -118.2143)
  line L622 (134.3483, -104.2443) -> (135.3288, -104.2443)
  line L623 (135.3288, -104.2443) -> (135.3288, -118.2143)
  line L624 (135.3288, -118.2143) -> (134.3483, -118.2143)
  line L625 (130.8482, -118.2143) -> (125.8393, -118.2143)
  line L626 (122.3392, -118.2143) -> (121.3588, -118.2143)
  line L627 (121.3588, -118.2143) -> (121.3588, -104.2443)
  line L628 (121.3588, -104.2443) -> (122.3392, -104.2443)
  line L629 (125.8393, -104.2443) -> (130.8482, -104.2443)
  line L630 (130.8482, -79.619) -> (134.3483, -79.619)
  line L631 (134.3483, -95.2146) -> (130.8482, -95.2146)
  line L632 (125.8393, -95.2146) -> (122.3392, -95.2146)
  line L633 (122.3392, -79.619) -> (125.8393, -79.619)
  line L634 (130.8482, -79.619) -> (130.8482, -80.4318)
  line L635 (130.8482, -94.4018) -> (130.8482, -95.2146)
  line L636 (125.8393, -95.2146) -> (125.8393, -94.4018)
  line L637 (125.8393, -80.4318) -> (125.8393, -79.619)
  line L638 (125.8393, -94.4018) -> (125.8393, -95.2146)
  line L639 (125.8393, -95.2146) -> (122.3392, -95.2146)
  line L640 (122.3392, -95.2146) -> (122.3392, -94.4018)
  line L641 (122.3392, -80.4318) -> (122.3392, -79.619)
  line L642 (122.3392, -79.619) -> (125.8393, -79.619)
  line L643 (125.8393, -79.619) -> (125.8393, -80.4318)
  line L644 (130.8482, -80.4318) -> (130.8482, -79.619)
  line L645 (130.8482, -79.619) -> (134.3483, -79.619)
  line L646 (134.3483, -79.619) -> (134.3483, -80.4318)
  line L647 (134.3483, -94.4018) -> (134.3483, -95.2146)
  line L648 (134.3483, -95.2146) -> (130.8482, -95.2146)
  line L649 (130.8482, -95.2146) -> (130.8482, -94.4018)
  line L650 (134.3483, -80.4318) -> (135.3288, -80.4318)
  line L651 (135.3288, -80.4318) -> (135.3288, -94.4018)
  line L652 (135.3288, -94.4018) -> (134.3483, -94.4018)
  line L653 (130.8482, -94.4018) -> (125.8393, -94.4018)
  line L654 (122.3392, -94.4018) -> (121.3588, -94.4018)
  line L655 (121.3588, -94.4018) -> (121.3588, -80.4318)
  line L656 (121.3588, -80.4318) -> (122.3392, -80.4318)
  line L657 (125.8393, -80.4318) -> (130.8482, -80.4318)
  line L658 (149.8982, -291.5503) -> (153.3983, -291.5503)
  line L659 (153.3983, -307.1459) -> (149.8982, -307.1459)
  line L660 (144.8893, -307.1459) -> (141.3892, -307.1459)
  line L661 (141.3892, -291.5503) -> (144.8893, -291.5503)
  line L662 (149.8982, -291.5503) -> (149.8982, -292.3631)
  line L663 (149.8982, -306.3331) -> (149.8982, -307.1459)
  line L664 (144.8893, -307.1459) -> (144.8893, -306.3331)
  line L665 (144.8893, -292.3631) -> (144.8893, -291.5503)
  line L666 (144.8893, -306.3331) -> (144.8893, -307.1459)
  line L667 (144.8893, -307.1459) -> (141.3892, -307.1459)
  line L668 (141.3892, -307.1459) -> (141.3892, -306.3331)
  line L669 (141.3892, -292.3631) -> (141.3892, -291.5503)
  line L670 (141.3892, -291.5503) -> (144.8893, -291.5503)
  line L671 (144.8893, -291.5503) -> (144.8893, -292.3631)
  line L672 (149.8982, -292.3631) -> (149.8982, -291.5503)
  line L673 (149.8982, -291.5503) -> (153.3983, -291.5503)
  line L674 (153.3983, -291.5503) -> (153.3983, -292.3631)
  line L675 (153.3983, -306.3331) -> (153.3983, -307.1459)
  line L676 (153.3983, -307.1459) -> (149.8982, -307.1459)
  line L677 (149.8982, -307.1459) -> (149.8982, -306.3331)
  line L678 (153.3983, -292.3631) -> (154.3788, -292.3631)
  line L679 (154.3788, -292.3631) -> (154.3788, -306.3331)
  line L680 (154.3788, -306.3331) -> (153.3983, -306.3331)
  line L681 (149.8982, -306.3331) -> (144.8893, -306.3331)
  line L682 (141.3892, -306.3331) -> (140.4088, -306.3331)
  line L683 (140.4088, -306.3331) -> (140.4088, -292.3631)
  line L684 (140.4088, -292.3631) -> (141.3892, -292.3631)
  line L685 (144.8893, -292.3631) -> (149.8982, -292.3631)
  line L686 (149.8982, -117.719) -> (153.3983, -117.719)
  line L687 (153.3983, -133.3146) -> (149.8982, -133.3146)
  line L688 (144.8893, -133.3146) -> (141.3892, -133.3146)
  line L689 (141.3892, -117.719) -> (144.8893, -117.719)
  line L690 (149.8982, -117.719) -> (149.8982, -118.5318)
  line L691 (149.8982, -132.5018) -> (149.8982, -133.3146)
  line L692 (144.8893, -133.3146) -> (144.8893, -132.5018)
  line L693 (144.8893, -118.5318) -> (144.8893, -117.719)
  line L694 (144.8893, -132.5018) -> (144.8893, -133.3146)
  line L695 (144.8893, -133.3146) -> (141.3892, -133.3146)
  line L696 (141.3892, -133.3146) -> (141.3892, -132.5018)
  line L697 (141.3892, -118.5318) -> (141.3892, -117.719)
  line L698 (141.3892, -117.719) -> (144.8893, -117.719)
  line L699 (144.8893, -117.719) -> (144.8893, -118.5318)
  line L700 (149.8982, -118.5318) -> (149.8982, -117.719)
  line L701 (149.8982, -117.719) -> (153.3983, -117.719)
  line L702 (153.3983, -117.719) -> (153.3983, -118.5318)
  line L703 (153.3983, -132.5018) -> (153.3983, -133.3146)
  line L704 (153.3983, -133.3146) -> (149.8982, -133.3146)
  line L705 (149.8982, -133.3146) -> (149.8982, -132.5018)
  line L706 (153.3983, -118.5318) -> (154.3788, -118.5318)
  line L707 (154.3788, -118.5318) -> (154.3788, -132.5018)
  line L708 (154.3788, -132.5018) -> (153.3983, -132.5018)
  line L709 (149.8982, -132.5018) -> (144.8893, -132.5018)
  line L710 (141.3892, -132.5018) -> (140.4088, -132.5018)
  line L711 (140.4088, -132.5018) -> (140.4088, -118.5318)
  line L712 (140.4088, -118.5318) -> (141.3892, -118.5318)
  line L713 (144.8893, -118.5318) -> (149.8982, -118.5318)
  line L714 (149.8982, -136.769) -> (153.3983, -136.769)
  line L715 (153.3983, -152.3646) -> (149.8982, -152.3646)
  line L716 (144.8893, -152.3646) -> (141.3892, -152.3646)
  line L717 (141.3892, -136.769) -> (144.8893, -136.769)
  line L718 (149.8982, -136.769) -> (149.8982, -137.5818)
  line L719 (149.8982, -151.5518) -> (149.8982, -152.3646)
  line L720 (144.8893, -152.3646) -> (144.8893, -151.5518)
  line L721 (144.8893, -137.5818) -> (144.8893, -136.769)
  line L722 (144.8893, -151.5518) -> (144.8893, -152.3646)
  line L723 (144.8893, -152.3646) -> (141.3892, -152.3646)
  line L724 (141.3892, -152.3646) -> (141.3892, -151.5518)
  line L725 (141.3892, -137.5818) -> (141.3892, -136.769)
  line L726 (141.3892, -136.769) -> (144.8893, -136.769)
  line L727 (144.8893, -136.769) -> (144.8893, -137.5818)
  line L728 (149.8982, -137.5818) -> (149.8982, -136.769)
  line L729 (149.8982, -136.769) -> (153.3983, -136.769)
  line L730 (153.3983, -136.769) -> (153.3983, -137.5818)
  line L731 (153.3983, -151.5518) -> (153.3983, -152.3646)
  line L732 (153.3983, -152.3646) -> (149.8982, -152.3646)
  line L733 (149.8982, -152.3646) -> (149.8982, -151.5518)
  line L734 (153.3983, -137.5818) -> (154.3788, -137.5818)
  line L735 (154.3788, -137.5818) -> (154.3788, -151.5518)
  line L736 (154.3788, -151.5518) -> (153.3983, -151.5518)
  line L737 (149.8982, -151.5518) -> (144.8893, -151.5518)
  line L738 (141.3892, -151.5518) -> (140.4088, -151.5518)
  line L739 (140.4088, -151.5518) -> (140.4088, -137.5818)
  line L740 (140.4088, -137.5818) -> (141.3892, -137.5818)
  line L741 (144.8893, -137.5818) -> (149.8982, -137.5818)
  line L742 (149.8982, -155.819) -> (153.3983, -155.819)
  line L743 (153.3983, -171.4146) -> (149.8982, -171.4146)
  line L744 (144.8893, -171.4146) -> (141.3892, -171.4146)
  line L745 (141.3892, -155.819) -> (144.8893, -155.819)
  line L746 (149.8982, -155.819) -> (149.8982, -156.6318)
  line L747 (149.8982, -170.6018) -> (149.8982, -171.4146)
  line L748 (144.8893, -171.4146) -> (144.8893, -170.6018)
  line L749 (144.8893, -156.6318) -> (144.8893, -155.819)
  line L750 (144.8893, -170.6018) -> (144.8893, -171.4146)
  line L751 (144.8893, -171.4146) -> (141.3892, -171.4146)
  line L752 (141.3892, -171.4146) -> (141.3892, -170.6018)
  line L753 (141.3892, -156.6318) -> (141.3892, -155.819)
  line L754 (141.3892, -155.819) -> (144.8893, -155.819)
  line L755 (144.8893, -155.819) -> (144.8893, -156.6318)
  line L756 (149.8982, -156.6318) -> (149.8982, -155.819)
  line L757 (149.8982, -155.819) -> (153.3983, -155.819)
  line L758 (153.3983, -155.819) -> (153.3983, -156.6318)
  line L759 (153.3983, -170.6018) -> (153.3983, -171.4146)
  line L760 (153.3983, -171.4146) -> (149.8982, -171.4146)
  line L761 (149.8982, -171.4146) -> (149.8982, -170.6018)
  line L762 (153.3983, -156.6318) -> (154.3788, -156.6318)
  line L763 (154.3788, -156.6318) -> (154.3788, -170.6018)
  line L764 (154.3788, -170.6018) -> (153.3983, -170.6018)
  line L765 (149.8982, -170.6018) -> (144.8893, -170.6018)
  line L766 (141.3892, -170.6018) -> (140.4088, -170.6018)
  line L767 (140.4088, -170.6018) -> (140.4088, -156.6318)
  line L768 (140.4088, -156.6318) -> (141.3892, -156.6318)
  line L769 (144.8893, -156.6318) -> (149.8982, -156.6318)
  line L770 (149.8982, -174.869) -> (153.3983, -174.869)
  line L771 (153.3983, -190.4646) -> (149.8982, -190.4646)
  line L772 (144.8893, -190.4646) -> (141.3892, -190.4646)
  line L773 (141.3892, -174.869) -> (144.8893, -174.869)
  line L774 (149.8982, -174.869) -> (149.8982, -175.6818)
  line L775 (149.8982, -189.6518) -> (149.8982, -190.4646)
  line L776 (144.8893, -190.4646) -> (144.8893, -189.6518)
  line L777 (144.8893, -175.6818) -> (144.8893, -174.869)
  line L778 (144.8893, -189.6518) -> (144.8893, -190.4646)
  line L779 (144.8893, -190.4646) -> (141.3892, -190.4646)
  line L780 (141.3892, -190.4646) -> (141.3892, -189.6518)
  line L781 (141.3892, -175.6818) -> (141.3892, -174.869)
  line L782 (141.3892, -174.869) -> (144.8893, -174.869)
  line L783 (144.8893, -174.869) -> (144.8893, -175.6818)
  line L784 (149.8982, -175.6818) -> (149.8982, -174.869)
  line L785 (149.8982, -174.869) -> (153.3983, -174.869)
  line L786 (153.3983, -174.869) -> (153.3983, -175.6818)
  line L787 (153.3983, -189.6518) -> (153.3983, -190.4646)
  line L788 (153.3983, -190.4646) -> (149.8982, -190.4646)
  line L789 (149.8982, -190.4646) -> (149.8982, -189.6518)
  line L790 (153.3983, -175.6818) -> (154.3788, -175.6818)
  line L791 (154.3788, -175.6818) -> (154.3788, -189.6518)
  line L792 (154.3788, -189.6518) -> (153.3983, -189.6518)
  line L793 (149.8982, -189.6518) -> (144.8893, -189.6518)
  line L794 (141.3892, -189.6518) -> (140.4088, -189.6518)
  line L795 (140.4088, -189.6518) -> (140.4088, -175.6818)
  line L796 (140.4088, -175.6818) -> (141.3892, -175.6818)
  line L797 (144.8893, -175.6818) -> (149.8982, -175.6818)
  line L798 (149.8982, -193.919) -> (153.3983, -193.919)
  line L799 (153.3983, -209.5146) -> (149.8982, -209.5146)
  line L800 (144.8893, -209.5146) -> (141.3892, -209.5146)
  line L801 (141.3892, -193.919) -> (144.8893, -193.919)
  line L802 (149.8982, -193.919) -> (149.8982, -194.7318)
  line L803 (149.8982, -208.7018) -> (149.8982, -209.5146)
  line L804 (144.8893, -209.5146) -> (144.8893, -208.7018)
  line L805 (144.8893, -194.7318) -> (144.8893, -193.919)
  line L806 (144.8893, -208.7018) -> (144.8893, -209.5146)
  line L807 (144.8893, -209.5146) -> (141.3892, -209.5146)
  line L808 (141.3892, -209.5146) -> (141.3892, -208.7018)
  line L809 (141.3892, -194.7318) -> (141.3892, -193.919)
  line L810 (141.3892, -193.919) -> (144.8893, -193.919)
  line L811 (144.8893, -193.919) -> (144.8893, -194.7318)
  line L812 (149.8982, -194.7318) -> (149.8982, -193.919)
  line L813 (149.8982, -193.919) -> (153.3983, -193.919)
  line L814 (153.3983, -193.919) -> (153.3983, -194.7318)
  line L815 (153.3983, -208.7018) -> (153.3983, -209.5146)
  line L816 (153.3983, -209.5146) -> (149.8982, -209.5146)
  line L817 (149.8982, -209.5146) -> (149.8982, -208.7018)
  line L818 (153.3983, -194.7318) -> (154.3788, -194.7318)